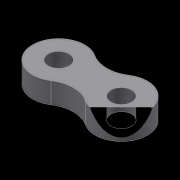
# Autodesk Inventor part: ChainLink
Saved by Autodesk Inventor 2015 (Build 190159000, 159)
## iProperties
Created: 2015-07-29
Part Number: ChainLink
Material: Generic
Document SubType Name: Modeling
Designer: Val
Density: 1 g/cm^3
Appearance: Default
Author: Val
Autodesk Inventor part; units mm, degrees
ref_plane "YZ Plane" through (0, 0, 0) normal (1, 0, 0) x (0, 1, 0)
ref_plane "XZ Plane" through (0, 0, 0) normal (0, 1, 0) x (-1, 0, 0)
ref_plane "XY Plane" through (0, 0, 0) normal (0, 0, 1) x (1, 0, 0)
sketch "Body" plane through (0, 0, 0) normal (0, 0, 1) x (1, 0, 0)
  circle A0 centre (0, 0) radius 0.5
  line L0 (0, 0) -> (3, 0) construction
  circle A1 centre (3, 0) radius 0.5
  arc A2 (0.6818, 1.0477) -> (0.6818, -1.0477) centre (0, 0) ccw
  arc A3 (2.3182, -1.0477) -> (2.3182, 1.0477) centre (3, 0) ccw
  arc A4 (0.6818, 1.0477) -> (2.3182, 1.0477) centre (1.5, 2.3049) ccw
  arc A5 (2.3182, -1.0477) -> (0.6818, -1.0477) centre (1.5, -2.3049) ccw
  dimension "d0" = 1
  dimension "d1" = 3
  dimension "d2" = 1
  dimension "d3" = 2.5
  dimension "d5" = 1.5
  constraints: 8 point on circle, 6 centre point, 4 coincident, 3 symmetric about line, 2 end point, 2 tangent, 1 equal radius, 1 horizontal, 1 other
  measures "d0" diameter of A0
  measures "d1" distance of L0.start L0.end
  measures "d2" diameter of A1
  measures "d3" diameter of A2
  measures "d5" radius of A4
extrude "BodyFeature" add sketch "Body" along normal blind 1
